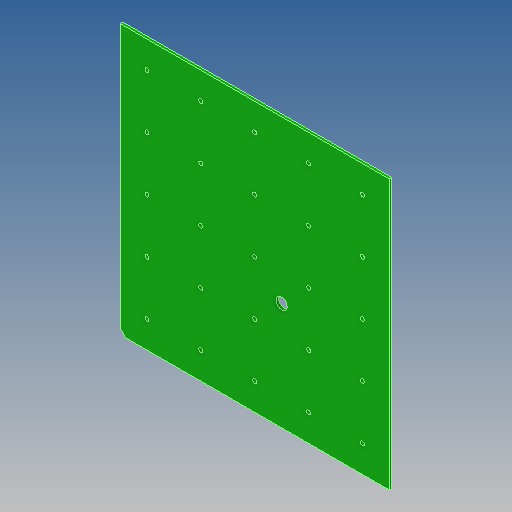
# Autodesk Inventor part: PCB RGB
Saved by Autodesk Inventor 2018.2 (Build 222227000, 227)
## iProperties
Created: 2017-12-19
Part Number: PCB RGB
Material: Generic
Document SubType Name: Modeling
Designer: Igor
Density: 1 g/cm^3
Appearance: Dark Green
Project: COMMON
Description: PCB RGB
Vendor: MCMASTER
ALTERED ITEM DESCRIPTION: N/A
ALTERED ITEM PART NUMBER: N/A
ALTERED ITEM VENDOR: N/A
DESIGN DEPARTMENT: HHMI: JRC - ID&F
LAB/DEPT: COMMON
REQUESTING SCIENTIST: COMMON
SPECIAL FINISH: NONE
SURFACE ROUGHNESS: N/A
Author: Igor
Revision Number: -
Autodesk Inventor part; units mm, degrees
ref_plane "YZ Plane" through (0, 0, 0) normal (1, 0, 0) x (0, 1, 0)
ref_plane "XZ Plane" through (0, 0, 0) normal (0, 1, 0) x (-1, 0, 0)
ref_plane "XY Plane" through (0, 0, 0) normal (0, 0, 1) x (1, 0, 0)
sketch "Sketch1" plane through (0, 0, 0) normal (0, 0, 1) x (1, 0, 0)
  line L0 (0, 0) -> (152.4, 0)
  line L1 (152.4, 0) -> (152.4, 152.4)
  line L2 (152.4, 152.4) -> (0, 152.4)
  line L3 (0, 152.4) -> (0, 0)
  line L4 (0, 3.175) -> (3.175, 0)
  circle A0 centre (15.24, 15.24) radius 1.143
  circle A1 centre (45.72, 15.24) radius 1.143
  circle A2 centre (76.2, 15.24) radius 1.143
  circle A3 centre (106.68, 15.24) radius 1.143
  circle A4 centre (137.16, 15.24) radius 1.143
  circle A5 centre (15.24, 45.72) radius 1.143
  circle A6 centre (45.72, 45.72) radius 1.143
  circle A7 centre (76.2, 45.72) radius 1.143
  circle A8 centre (106.68, 45.72) radius 1.143
  circle A9 centre (137.16, 45.72) radius 1.143
  circle A10 centre (15.24, 76.2) radius 1.143
  circle A11 centre (45.72, 76.2) radius 1.143
  circle A12 centre (76.2, 76.2) radius 1.143
  circle A13 centre (106.68, 76.2) radius 1.143
  circle A14 centre (137.16, 76.2) radius 1.143
  circle A15 centre (15.24, 106.68) radius 1.143
  circle A16 centre (45.72, 106.68) radius 1.143
  circle A17 centre (76.2, 106.68) radius 1.143
  circle A18 centre (106.68, 106.68) radius 1.143
  circle A19 centre (137.16, 106.68) radius 1.143
  circle A20 centre (15.24, 137.16) radius 1.143
  circle A21 centre (45.72, 137.16) radius 1.143
  circle A22 centre (76.2, 137.16) radius 1.143
  circle A23 centre (106.68, 137.16) radius 1.143
  circle A24 centre (137.16, 137.16) radius 1.143
  circle A25 centre (91.44, 60.96) radius 3.175
  dimension "d0" = 152.4
  dimension "d1" = 152.4
  dimension "d2" = 3.175
  dimension "d3" = 3.175
  dimension "d4" = 2.286
  dimension "d5" = 15.24
  dimension "d6" = 15.24
  dimension "d9" = 30.48
  dimension "d12" = 30.48
  dimension "d15" = 91.44
  dimension "d16" = 60.96
  dimension "d17" = 6.35
  constraints: 26 centre point, 10 end point, 2 horizontal, 2 parallel, 2 point on line, 1 perpendicular, 1 vertical, 48 other
  measures "d0" distance between parallel lines of L0 L2
  measures "d1" distance of L0.start L0.end
  measures "d2" distance from line of L4.end L3
  measures "d3" distance from line of L4.start L0
  measures "d4" diameter of A0
  measures "d5" distance from line of A0.centre L3
  measures "d6" distance from line of A0.centre L0
  measures "d9" distance of A0.centre A1.centre
  measures "d12" distance of A0.centre A5.centre
  measures "d15" distance from line of L3 A25.centre
  measures "d16" distance from line of L0 A25.centre
  measures "d17" diameter of A25
extrude "Extrusion1" add sketch "Sketch1" against normal blind 1.5 contours L4 L3 L2 L1 L0
equation "\"d3\" = d2"
body "Solid1"
